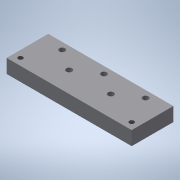
# Autodesk Inventor part: AgarMouldBottomV3
Saved by Autodesk Inventor 2021 (Build 250183000, 183)
## iProperties
Created: 2013-04-25
Part Number: AgarMouldBottomV3
Material: Generic
Document SubType Name: Modeling
Designer: 120pa
Density: 1 g/cm^3
Appearance: Default
Author: 120pa
Autodesk Inventor part; units mm, degrees
ref_plane "YZ Plane" through (0, 0, 0) normal (1, 0, 0) x (0, 1, 0)
ref_plane "XZ Plane" through (0, 0, 0) normal (0, 1, 0) x (-1, 0, 0)
ref_plane "XY Plane" through (0, 0, 0) normal (0, 0, 1) x (1, 0, 0)
sketch "Sketch1" plane through (0, 0, 0) normal (0, 1, 0) x (-1, 0, 0)
  line L0 (31.8795, -5.6386) -> (-58.1205, -5.6386)
  line L1 (-58.1205, -5.6386) -> (-58.1205, 24.3614)
  line L2 (-58.1205, 24.3614) -> (31.8795, 24.3614)
  line L3 (31.8795, 24.3614) -> (31.8795, -5.6386)
  point P0 (0, 0)
  dimension "d0" = 90
  dimension "d5" = 30
  constraints: 8 end point, 2 parallel, 1 horizontal, 1 perpendicular
  measures "d0" distance of L1.end L2.end
  measures "d5" distance of L2.end L0.start
extrude "Extrusion1" add sketch "Sketch1" along normal blind 10
sketch "Sketch2" plane through (0, 10, 0) normal (0, 1, 0) x (1, 0, 0)
  line L0 (58.1205, 5.6386) -> (-31.8795, 5.6386) projected
  line L1 (-31.8795, 5.6386) -> (-31.8795, -24.3614) projected
  circle A0 centre (-16.8795, 0.6386) radius 2.05
  circle A1 centre (13.1205, 0.6386) radius 2.05
  circle A2 centre (43.1205, 0.6386) radius 2.05
  point P0 (0, 0)
  dimension "d8" = 4.1
  dimension "d10" = 4.1
  dimension "d11" = 4.1
  dimension "d12" = 5
  dimension "d13" = 5
  dimension "d14" = 5
  dimension "d15" = 15
  dimension "d16" = 30
  dimension "d17" = 30
  constraints: 3 centre point
  measures "d8" diameter of A0
  measures "d10" diameter of A1
  measures "d11" diameter of A2
  measures "d12" distance from line of L0 A0.centre
  measures "d13" distance from line of L0 A1.centre
  measures "d14" distance from line of L0 A2.centre
  measures "d15" distance from line of L1 A0.centre
  measures "d16" distance of A1.centre A0.centre
  measures "d17" distance of A2.centre A1.centre
extrude "Extrusion2" cut sketch "Sketch2" against normal blind 10
sketch "Sketch4" plane through (0, 0, 0) normal (0, -1, 0) x (1, 0, 0)
  circle A0 centre (13.1205, -0.6386) radius 2.05 projected
  circle A1 centre (-16.8795, -0.6386) radius 2.05 projected
  circle A2 centre (43.1205, -0.6386) radius 2.05 projected
  circle A3 centre (-16.8795, -0.6386) radius 3.5
  circle A4 centre (13.1205, -0.6386) radius 3.5
  circle A5 centre (43.1205, -0.6386) radius 3.5
  point P0 (0, 0)
  dimension "d26" = 7
  dimension "d28" = 7
  dimension "d29" = 7
  constraints: 3 centre point, 3 coincident
  measures "d26" diameter of A3
  measures "d28" diameter of A4
  measures "d29" diameter of A5
extrude "Extrusion4" cut sketch "Sketch4" against normal blind 4.5
sketch "Sketch5" plane through (0, 0, 0) normal (0, -1, 0) x (1, 0, 0)
  line L0 (58.1205, -5.6386) -> (58.1205, 24.3614) projected
  line L1 (58.1205, 24.3614) -> (-31.8795, 24.3614) projected
  line L2 (-31.8795, 24.3614) -> (-31.8795, -5.6386) projected
  circle A0 centre (-1.8795, 9.3614) radius 2.1
  circle A1 centre (28.1205, 9.3614) radius 2.1
  point P0 (0, 0)
  dimension "d32" = 4.2
  dimension "d34" = 4.2
  dimension "d35" = 30
  dimension "d36" = 30
  dimension "d37" = 15
  dimension "d38" = 15
  constraints: 2 centre point
  measures "d32" diameter of A0
  measures "d34" diameter of A1
  measures "d35" distance from line of L2 A0.centre
  measures "d36" distance from line of L0 A1.centre
  measures "d37" distance from line of L1 A0.centre
  measures "d38" distance from line of L1 A1.centre
extrude "Extrusion5" cut sketch "Sketch5" against normal blind 10
sketch "Sketch6" plane through (0, 0, 0) normal (0, -1, 0) x (1, 0, 0)
  circle A0 centre (-1.8795, 9.3614) radius 2.1 projected
  circle A1 centre (28.1205, 9.3614) radius 2.1 projected
  circle A2 centre (-1.8795, 9.3614) radius 3.5
  circle A3 centre (28.1205, 9.3614) radius 3.5
  point P0 (0, 0)
  dimension "d41" = 7
  dimension "d43" = 7
  constraints: 2 centre point, 2 coincident
  measures "d41" diameter of A2
  measures "d43" diameter of A3
extrude "Extrusion6" cut sketch "Sketch6" against normal blind 4.5
sketch "Sketch8" plane through (0, 10, 0) normal (0, 1, 0) x (1, 0, 0)
  line L0 (-31.8795, 5.6386) -> (-31.8795, -24.3614) projected
  line L1 (-31.8795, -24.3614) -> (-26.8795, -24.3614)
  line L2 (-26.8795, -24.3614) -> (-26.8795, -19.3614)
  line L3 (-26.8795, -19.3614) -> (-31.8795, -19.3614)
  line L4 (-31.8795, -19.3614) -> (-31.8795, -24.3614)
  line L5 (-31.8795, -24.3614) -> (58.1205, -24.3614) projected
  line L6 (58.1205, -24.3614) -> (53.1205, -24.3614)
  line L7 (53.1205, -24.3614) -> (53.1205, -19.3614)
  line L8 (53.1205, -19.3614) -> (58.1205, -19.3614)
  line L9 (58.1205, -19.3614) -> (58.1205, -24.3614)
  point P0 (0, 0)
  dimension "d58" = 5
  dimension "d59" = 5
  dimension "d62" = 5
  dimension "d63" = 5
  constraints: 16 end point, 4 parallel, 2 horizontal, 2 perpendicular
  measures "d58" distance of L3.end L2.end
  measures "d59" distance of L2.end L1.end
  measures "d62" distance of L7.end L8.end
  measures "d63" distance of L6.end L7.end
hole "Hole1" at (-26.8795, 10, 19.3614) at (53.1205, 10, 19.3614) direction (0, -1, 0) diameter 3.302 depth 12.3 thread size "8-32 UNC" class "2B" standard "ANSI Unified Screw Threads"
equation "\"d10\" = d8"
equation "\"d11\" = d8"
equation "\"d13\" = d12"
equation "\"d14\" = d12"
equation "\"d28\" = d26"
equation "\"d29\" = d26"
body "Solid1"
